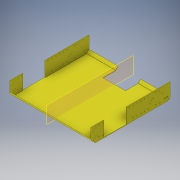
# Autodesk Inventor part: SheetBottomFloorV01_sheet_metal
Saved by Autodesk Inventor 2016 SP1 (Build 200210100, 210)
## iProperties
Created: 2016-02-09
Part Number: SheetBottomFloorV01_sheet_metal
Material: Aluminum 6061
Document SubType Name: Sheet Metal
Designer: steele
Density: 2.7 g/cm^3
Appearance: Canary
Sheet Metal Rule: Default
Author: steele
Autodesk Inventor part; units mm, degrees
ref_plane "XZ Plane" through (0, 0, 0) normal (0, 1, 0) x (-1, 0, 0)
ref_plane "XY Plane" through (0, 0, 0) normal (0, 0, 1) x (1, 0, 0)
sketch "Sketch1" plane through (0, 0, 0) normal (0, 0, 1) x (1, 0, 0)
  line L0 (0, 0) -> (-273.05, 0)
  line L1 (-273.05, 0) -> (-273.05, 101.6)
  line L2 (-273.05, 101.6) -> (-269.875, 101.6)
  line L3 (-269.875, 101.6) -> (-269.875, 3.175)
  line L4 (0, 0) -> (0, 3.175) construction
  line L5 (0, 3.175) -> (-269.875, 3.175)
  line L6 (0, 0) -> (273.05, 0)
  line L7 (273.05, 0) -> (273.05, 101.6)
  line L8 (273.05, 101.6) -> (269.875, 101.6)
  line L9 (269.875, 101.6) -> (269.875, 3.175)
  line L10 (0, 3.175) -> (269.875, 3.175)
  dimension "d0" = 101.6
  dimension "d1" = 273.05
  dimension "d2" = 3.175
  dimension "d4" = 3.175
  constraints: 22 end point, 4 symmetric about line, 2 horizontal, 2 perpendicular, 1 parallel, 1 vertical
  measures "d0" distance of L0.end L1.end
  measures "d1" distance of L0.start L0.end
  measures "d2" distance between parallel lines of L1 L3
  measures "d4" distance of L0.start L4.end
extrude "Extrusion1" add sketch "Sketch1" along normal mid plane 527.05
fillet "Fillet1" radius 0.7937 2 edges at (-269.875, 3.175, 0) (269.875, 3.175, 0)
sketch "Sketch5" plane through (-269.875, 101.6, 263.525) normal (1, 0, 0) x (0, 0, -1)
  circle A0 centre (12.7, -30.1625) radius 2.5527 projected
  circle A1 centre (22.225, -20.6375) radius 2.5527 projected
  circle A2 centre (31.75, -11.1125) radius 2.5527 projected
  circle A3 centre (50.8, -11.1125) radius 3.3782 projected
  circle A4 centre (76.2, -11.1125) radius 3.7287 projected
  circle A5 centre (12.7, -84.1375) radius 2.667 projected
  circle A6 centre (22.225, -74.6125) radius 2.667 projected
  circle A7 centre (31.75, -65.0875) radius 2.5527 projected
  circle A8 centre (50.8, -77.7875) radius 3.8163 projected
  circle A9 centre (76.2, -84.1375) radius 3.3782 projected
  circle A10 centre (101.4806, -88.9127) radius 3.3782 projected
  circle A11 centre (212.631, -88.9127) radius 3.3782 projected
  circle A12 centre (228.6, -84.1375) radius 3.7287 projected
  circle A13 centre (279.4, -81.5975) radius 3.8163 projected
  circle A14 centre (228.6, -11.1125) radius 3.3782 projected
  circle A15 centre (254, -11.1125) radius 3.7287 projected
  circle A16 centre (279.4, -11.1125) radius 3.3782 projected
  circle A17 centre (304.8, -11.1125) radius 3.3782 projected
  circle A18 centre (330.2, -11.1125) radius 3.7287 projected
  circle A19 centre (355.6, -11.1125) radius 3.3782 projected
  circle A20 centre (381, -11.1125) radius 3.3782 projected
  circle A21 centre (431.8, -11.1125) radius 3.7287 projected
  circle A22 centre (454.025, -14.2875) radius 3.8163 projected
  circle A23 centre (508, -77.7875) radius 3.8163 projected
  circle A24 centre (457.2, -84.1375) radius 3.3782 projected
  circle A25 centre (431.8, -84.1375) radius 3.7287 projected
  circle A26 centre (475.0995, -39.081) radius 3.3782 projected
  circle A27 centre (412.75, -38.1) radius 2.5527 projected
  circle A28 centre (403.225, -47.625) radius 2.667 projected
  circle A29 centre (393.7, -57.15) radius 2.5527 projected
  circle A30 centre (381, -84.1375) radius 3.3782 projected
  circle A31 centre (355.6, -84.1375) radius 3.3782 projected
  circle A32 centre (330.2, -84.1375) radius 3.7287 projected
  circle A33 centre (304.8, -84.1375) radius 3.3782 projected
  circle A34 centre (492.125, -77.7875) radius 4.826 projected
  circle A35 centre (508, -77.7875) radius 5.2255 projected
  point P0 (263.525, -101.6)
extrude "Extrusion5" cut sketch "Sketch5" along normal through all both and the other way through all
sketch "Sketch7" plane through (-269.875, 101.6, 263.525) normal (1, 0, 0) x (0, 0, -1)
  line L0 (0, 0) -> (527.05, 0) projected
  line L1 (82.55, 0) -> (234.95, 0)
  line L2 (234.95, 0) -> (234.95, -96.8375)
  line L3 (234.95, -96.8375) -> (82.55, -96.8375)
  line L4 (82.55, -96.8375) -> (82.55, 0)
  line L5 (0, -101.6) -> (527.05, -101.6) projected
  line L6 (0, 0) -> (0, -101.6) projected
  point P0 (263.525, -101.6)
  dimension "d26" = 4.7625
  dimension "d27" = 82.55
  dimension "d28" = 234.95
  constraints: 8 end point, 2 parallel, 1 horizontal, 1 perpendicular, 1 point on line
  measures "d26" distance between parallel lines of L5 L3
  measures "d27" distance between parallel lines of L6 L4
  measures "d28" distance between parallel lines of L2 L6
extrude "Extrusion6" cut sketch "Sketch7" along normal through all both and the other way through all
sketch "Sketch8" plane through (-269.0813, 3.175, -263.525) normal (0, 1, 0) x (1, 0, 0)
  line L0 (-0.7937, 0) -> (-0.7937, -527.05) projected
  line L1 (-0.7937, -527.05) -> (538.3214, -527.05)
  line L2 (538.3214, -527.05) -> (538.3214, -501.65)
  line L3 (538.3214, -501.65) -> (-0.7937, -501.65)
  line L4 (-0.7937, -501.65) -> (-0.7937, -527.05)
  point P0 (269.0813, -263.525)
  dimension "d31" = 25.4
  constraints: 8 end point, 2 parallel, 1 horizontal, 1 perpendicular
  measures "d31" distance between parallel lines of L3 L1
extrude "Extrusion7" cut sketch "Sketch8" against normal through all
sketch "Sketch9" plane through (-269.875, 3.9687, 263.525) normal (1, 0, 0) x (0, 0, -1)
  line L0 (0, -3.9688) -> (527.05, -3.9688) projected
  line L1 (25.4, -3.9688) -> (0, 21.4312)
  line L2 (0, 97.6312) -> (0, -3.9688) projected
  line L3 (0, 21.4312) -> (0, 30.5124)
  line L4 (34.6319, -3.9688) -> (25.4, -3.9688)
  line L5 (0, 30.5124) -> (34.6319, -3.9688)
  point P0 (263.525, -3.9687)
  dimension "d34" = 25.4
  dimension "d35" = 45
  dimension "d36" = 0.125
  constraints: 8 end point, 4 point on line, 1 collinear
  measures "d34" distance from line of L1.start L2
  measures "d35" angle of L1 L0
  measures "d36" angle of L5 L1
extrude "Extrusion8" add sketch "Sketch9" along normal blind 539.75 contours L1 L2 L5 L0
sketch "Sketch10" plane through (-269.875, 3.9687, -263.525) normal (1, 0, 0) x (0, 0, -1)
  line L0 (-501.65, -3.9688) -> (-523.2125, 17.5937)
  line L1 (-527.05, 97.6312) -> (-527.05, -3.9688) projected
  line L2 (-527.05, -3.9688) -> (0, -3.9688) projected
  line L3 (-501.65, -3.9688) -> (-527.05, -3.9688)
  line L4 (-527.05, -3.9688) -> (-527.05, 21.4312)
  line L5 (-527.05, 21.4312) -> (-523.2125, 17.5937)
  point P0 (-263.525, -3.9687)
  dimension "d39" = 25.4
  dimension "d40" = 45
  constraints: 8 end point, 2 point on line, 1 collinear
  measures "d39" distance from line of L0.start L1
  measures "d40" angle of L0 L2
extrude "Extrusion9" cut sketch "Sketch10" along normal through all both and the other way through all
sketch "Sketch12" plane through (-269.875, 23.8125, -244.475) normal (1, 0, 0) x (0, 0, -1)
  circle A0 centre (0, 0) radius 4.2111
  point P0 (-244.475, -23.8125)
  constraints: 1 centre point
extrude "Extrusion10" cut sketch "Sketch12" along normal through all both and the other way through all
sketch "Sketch15" plane through (-269.875, 3.9687, -263.525) normal (1, 0, 0) x (0, 0, -1)
  line L0 (-101.6, -3.9687) -> (0, -3.9687) projected
  line L1 (0, -3.9687) -> (-15.875, -3.9687)
  line L2 (-15.875, -3.9687) -> (-15.875, -0.0063)
  line L3 (-15.875, -0.0063) -> (0, -0.0063)
  line L4 (0, -0.0063) -> (0, -3.9687)
  line L5 (0, -3.9687) -> (0, 97.6312) projected
  point P0 (-263.525, -3.9687)
  dimension "d51" = 15.875
  dimension "d54" = 3.9624
  constraints: 8 end point, 2 parallel, 1 horizontal, 1 perpendicular
  measures "d51" distance between parallel lines of L2 L4
  measures "d54" distance between parallel lines of L3 L0
extrude "Extrusion12" cut sketch "Sketch15" along normal through all both and the other way through all
sketch "Sketch16" plane through (-269.875, 3.9687, -263.525) normal (1, 0, 0) x (0, 0, -1)
  line L0 (-15.875, -0.0063) -> (-15.875, -3.9688) projected
  line L1 (-15.875, -3.9688) -> (0, 11.9063)
  line L2 (0, -0.0063) -> (0, 97.6312) projected
  line L3 (0, -0.0063) -> (-15.875, -0.0063) projected
  line L4 (-15.875, -0.0063) -> (0, 15.8687)
  line L5 (0, 15.8687) -> (0, 11.9063)
  line L6 (-15.875, -3.9688) -> (-15.875, -0.0063)
  point P0 (-263.525, -3.9687)
  dimension "d57" = 45
  constraints: 8 end point, 2 equal length, 2 point on line
  measures "d57" angle of L1 L0
extrude "Extrusion13" add sketch "Sketch16" along normal blind 539.75 contours L3 L1 L0 | L4 L2 L1 L3
sketch "Sketch17" plane through (-269.875, 4.7625, 28.575) normal (1, 0, 0) x (0, 0, -1)
  line L0 (292.1, -0.8001) -> (276.225, -0.8001) projected
  line L1 (276.225, -0.8001) -> (292.1, 15.0749)
  line L2 (292.1, -0.8001) -> (292.1, 96.8375) projected
  line L3 (276.225, -0.8001) -> (292.1, -0.8001)
  point P0 (28.575, -4.7625)
  dimension "d60" = 45
  constraints: 4 end point, 1 collinear, 1 point on line
  measures "d60" angle of L1 L0
extrude "Extrusion14" cut sketch "Sketch17" against normal through all
sketch "Sketch18" plane through (269.875, 3.9688, -263.525) normal (-1, 0, 0) x (0, 0, 1)
  line L0 (0, 11.9063) -> (11.9063, 0) projected
  line L1 (11.9063, 0) -> (0, 11.9063)
  line L2 (0, 0) -> (11.9063, 0) projected
  line L3 (11.9063, 0) -> (0, 0)
  line L4 (0, 0) -> (0, 11.9063) projected
  line L5 (0, 0) -> (0, 11.9063)
  point P0 (263.525, -3.9687)
  constraints: 6 end point, 2 collinear, 1 perpendicular
extrude "Extrusion15" cut sketch "Sketch18" against normal through all
sketch "Sketch14" plane through (-273.05, 0, -263.525) normal (0, -1, 0) x (1, 0, 0)
  line L0 (273.05, 263.525) -> (273.05, 0) construction
  line L1 (3.9687, 0) -> (542.1313, 0) construction
  line L2 (349.25, 101.6) -> (196.85, 101.6)
  line L3 (196.85, 101.6) -> (196.85, 0)
  line L4 (196.85, 0) -> (349.25, 0)
  line L5 (349.25, 0) -> (349.25, 101.6)
  line L6 (349.25, 101.6) -> (196.85, 0) construction
  line L7 (196.85, 101.6) -> (349.25, 0) construction
  line L8 (546.1, 0) -> (0, 0) projected
  point P0 (273.05, 50.8)
  dimension "d47" = 101.6
  dimension "d48" = 152.4
  constraints: 14 end point, 3 midpoint, 2 parallel, 2 perpendicular, 1 collinear, 1 point on line
  measures "d47" distance of L4.end L2.start
  measures "d48" distance of L2.start L2.end
extrude "Extrusion16" cut sketch "Sketch14" against normal blind 50.8
sketch "Sketch19" plane through (-269.875, 4.7625, 180.975) normal (0, 1, 0) x (1, 0, 0)
  line L0 (539.75, 0) -> (539.75, 152.4) projected
  line L1 (542.925, 0) -> (539.75, 0) projected
  line L2 (542.925, 152.4) -> (542.925, 0) projected
  line L3 (542.925, 152.4) -> (539.75, 152.4) projected
  line L4 (-3.175, 0) -> (-3.175, 152.4) projected
  line L5 (0, 0) -> (-3.175, 0) projected
  line L6 (0, 152.4) -> (0, 0) projected
  line L7 (0, 152.4) -> (-3.175, 152.4) projected
  line L8 (539.75, 152.4) -> (0, 152.4)
  line L9 (0, 152.4) -> (0, 0)
  line L10 (0, 0) -> (539.75, 0)
  line L11 (539.75, 0) -> (539.75, 152.4)
  point P0 (269.875, 180.975)
  constraints: 8 end point, 2 parallel, 1 horizontal, 1 perpendicular
extrude "Extrusion17" cut sketch "Sketch19" against normal up to surface (1.5875 mm away)
equation "\"BendRadius\" = Thickness"
equation "\"BendReliefWidth\" = Thickness"
equation "\"BendReliefDepth\" = 0.5 * Thickness"
equation "\"CornerReliefSize\" = 4 * Thickness"
equation "\"MinimumRemnant\" = 2 * Thickness"
equation "\"TransitionRadius\" = BendRadius"
equation "\"JacobiRadiusSize\" = Thickness"
equation "\"GapSize\" = Thickness"
equation "\"Thickness\" = 3.048"
body "Solid1"
